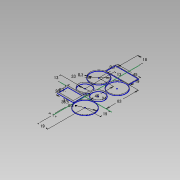
# Autodesk Inventor part: DoubleSlipHR_printbase
Saved by Autodesk Inventor 2021 (Build 250183000, 183)
## iProperties
Created: 2021-05-13
Part Number: DoubleSlipHR_printbase
Material: 一般
Document SubType Name: Modeling
Designer: kumagai
Density: 1 g/cm^3
Appearance: 既定
Author: kumagai
Autodesk Inventor part; units mm, degrees
ref_plane "YZ Plane" through (0, 0, 0) normal (1, 0, 0) x (0, 1, 0)
ref_plane "XZ Plane" through (0, 0, 0) normal (0, 1, 0) x (-1, 0, 0)
ref_plane "XY Plane" through (0, 0, 0) normal (0, 0, 1) x (1, 0, 0)
sketch "スケッチ1" plane through (0, 0, 0) normal (0, 1, 0) x (-1, 0, 0)
  line L0 (0, -106.27) -> (0, 61.52) projected
  line L1 (-52.02, 0) -> (49.27, 0) projected
  circle A0 centre (13, -13) radius 12
  circle A1 centre (13, -13) radius 12.3
  circle A2 centre (18, -45) radius 16.5
  circle A3 centre (18, -45) radius 16.8
  circle A4 centre (-13, -13) radius 12
  circle A5 centre (-13, -13) radius 12.3
  circle A6 centre (-18, -45) radius 16.5
  circle A7 centre (-18, -45) radius 16.8
  line L2 (32.6, 21.6) -> (1, 21.6)
  line L3 (1, 21.6) -> (1, 1)
  line L4 (1, 1) -> (32.6, 1)
  line L5 (32.6, 1) -> (32.6, 21.6)
  line L6 (32.3, 21.3) -> (1.3, 21.3)
  line L7 (1.3, 21.3) -> (1.3, 1.3)
  line L8 (1.3, 1.3) -> (32.3, 1.3)
  line L9 (32.3, 1.3) -> (32.3, 21.3)
  circle A8 centre (-19, 19) radius 18.55
  circle A9 centre (-19, 19) radius 18.25
  line L10 (22.8, -62.7) -> (-22.8, -62.7)
  line L11 (-22.8, -62.7) -> (-22.8, -82.3)
  line L12 (-22.8, -82.3) -> (22.8, -82.3)
  line L13 (22.8, -82.3) -> (22.8, -62.7)
  line L14 (22.5, -63) -> (-22.5, -63)
  line L15 (-22.5, -63) -> (-22.5, -82)
  line L16 (-22.5, -82) -> (22.5, -82)
  line L17 (22.5, -82) -> (22.5, -63)
  point P0 (0, 0)
  point P1 (0, -82.3)
  point P2 (0, -82)
  point P3 (0, -63)
  point P4 (0, -62.7)
  dimension "d0" = 24
  dimension "d1" = 0.3
  dimension "d2" = 13
  dimension "d3" = 13
  dimension "d4" = 33
  dimension "d5" = 0.3
  dimension "d6" = 18
  dimension "d7" = 45
  dimension "d12" = 0.3
  dimension "d13" = 1
  dimension "d14" = 1
  dimension "d15" = 20
  dimension "d16" = 31
  dimension "d17" = 0.3
  dimension "d18" = 36.5
  dimension "d19" = 19
  dimension "d20" = 19
  dimension "d25" = 0.3
  dimension "d26" = 19
  dimension "d27" = 63
  dimension "d28" = 45
  constraints: 32 end point, 10 centre point, 3 coincident, 11 other
  measures "d0" diameter of A0
  measures "d1" radial gap between concentric circles of A0 A1
  measures "d2" distance from line of L1 A0.centre
  measures "d3" distance from line of L0 A0.centre
  measures "d4" diameter of A2
  measures "d5" radial gap between concentric circles of A3 A2
  measures "d6" distance from line of L0 A2.centre
  measures "d7" distance from line of L1 A2.centre
  measures "d12" distance between parallel lines of L5 L9
  measures "d13" distance between parallel lines of L0 L3
  measures "d14" distance between parallel lines of L1 L4
  measures "d15" distance between parallel lines of L6 L8
  measures "d16" distance between parallel lines of L7 L9
  measures "d17" radial gap between concentric circles of A8 A9
  measures "d18" diameter of A9
  measures "d19" distance from line of L0 A8.centre
  measures "d20" distance from line of L1 A8.centre
  measures "d25" distance between parallel lines of L17 L13
  measures "d26" distance between parallel lines of L16 L14
  measures "d27" distance between parallel lines of L1 L14
  measures "d28" distance between parallel lines of L15 L17
extrude "押し出し1" add sketch "スケッチ1" along normal blind 2.8 contours A1 | A5
extrude "押し出し2" add sketch "スケッチ1" along normal blind 1.6 contours A3 | A7
extrude "押し出し3" add sketch "スケッチ1" along normal blind 3.2 contours L5 L4 L3 L2
extrude "押し出し4" add sketch "スケッチ1" along normal blind 1 contours A8
extrude "押し出し5" add sketch "スケッチ1" along normal blind 1 contours L12 L11 L10 L0 L14 L15 L16 | L0 L16 L17 L14 L10 L13 L12
